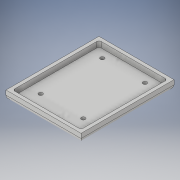
# Autodesk Inventor part: Motor_Node_top
Saved by Autodesk Inventor 2019.4 (Build 234330000, 330)
## iProperties
Created: 2019-12-12
Part Number: Motor_Node_top
Material: Generic
Document SubType Name: Modeling
Designer: Jorian Brusind
Density: 1 g/cm^3
Appearance: Default
Author: Jorian Brusind
Autodesk Inventor part; units mm, degrees
ref_plane "YZ Plane" through (0, 0, 0) normal (1, 0, 0) x (0, 1, 0)
ref_plane "XZ Plane" through (0, 0, 0) normal (0, 1, 0) x (-1, 0, 0)
ref_plane "XY Plane" through (0, 0, 0) normal (0, 0, 1) x (1, 0, 0)
sketch "Sketch1" plane through (0, 0, 0) normal (0, 1, 0) x (-1, 0, 0)
  line L0 (-33.5, 41.5) -> (33.5, 41.5)
  line L1 (33.5, 41.5) -> (33.5, -41.5)
  line L2 (33.5, -41.5) -> (-33.5, -41.5)
  line L3 (-33.5, -41.5) -> (-33.5, 41.5)
  line L4 (-33.5, 41.5) -> (33.5, -41.5) construction
  line L5 (33.5, 41.5) -> (-33.5, -41.5) construction
  point P0 (0, 0)
  dimension "d0" = 67
  dimension "d1" = 83
  constraints: 12 end point, 2 midpoint, 2 parallel, 1 horizontal, 1 perpendicular
  measures "d0" distance of L1.end L2.end
  measures "d1" distance of L0.end L1.end
extrude "Extrusion1" add sketch "Sketch1" along normal blind 3
sketch "Sketch2" plane through (0, 3, 0) normal (0, 1, 0) x (1, 0, 0)
  line L0 (-33.5, 41.5) -> (-33.5, -41.5) projected
  line L1 (33.5, 41.5) -> (-33.5, 41.5)
  line L2 (-33.5, 41.5) -> (-33.5, -41.5)
  line L3 (-33.5, -41.5) -> (33.5, -41.5)
  line L4 (33.5, -41.5) -> (33.5, 41.5)
  line L5 (33.5, 41.5) -> (-33.5, -41.5) construction
  line L6 (-33.5, 41.5) -> (33.5, -41.5) construction
  line L7 (30.5, 38.5) -> (-30.5, 38.5)
  line L8 (-30.5, 38.5) -> (-30.5, -38.5)
  line L9 (-30.5, -38.5) -> (30.5, -38.5)
  line L10 (30.5, -38.5) -> (30.5, 38.5)
  line L11 (30.5, 38.5) -> (-30.5, -38.5) construction
  line L12 (-30.5, 38.5) -> (30.5, -38.5) construction
  point P0 (0, 0)
  dimension "d4" = 61
  dimension "d5" = 77
  constraints: 24 end point, 4 midpoint, 4 parallel, 2 horizontal, 2 perpendicular
  measures "d4" distance of L9.end L8.end
  measures "d5" distance of L8.end L7.end
extrude "Extrusion2" add sketch "Sketch2" along normal blind 5
sketch "Sketch3" plane through (0, 3, 0) normal (0, 1, 0) x (1, 0, 0)
  circle A0 centre (18, 31) radius 1.75
  line L0 (-30.5, 38.5) -> (30.5, 38.5) projected
  line L1 (30.5, 38.5) -> (30.5, -38.5) projected
  circle A1 centre (18, -24) radius 1.75
  circle A2 centre (-20, 31) radius 1.75
  circle A3 centre (-20, -24) radius 1.75
  point P0 (0, 0)
  point P1 (30.5, -38.5)
  point P2 (26, 41.5)
  point P3 (26, -41.5)
  dimension "d8" = 3.5
  dimension "d9" = 7.5
  dimension "d10" = 12.5
  dimension "d13" = 55
  dimension "d16" = 38
  constraints: 4 centre point, 1 equal radius, 1 horizontal, 1 vertical alignment, 5 other
  measures "d8" diameter of A0
  measures "d9" distance from line of L0 A0.centre
  measures "d13" distance of A0.centre A1.centre
  measures "d16" distance of A0.centre A2.centre
extrude "Extrusion3" cut sketch "Sketch3" against normal blind 5
fillet "Fillet1" radius 4 4 edges at (33.5, 0, 0) (-33.5, 0, 0) (0, 0, 41.5) (0, 0, -41.5)
fillet "Fillet2" radius 2 4 edges at (-30.5, 5.5, -38.5) (30.5, 5.5, -38.5) (30.5, 5.5, 38.5) (-30.5, 5.5, 38.5)
body "Solid1"
